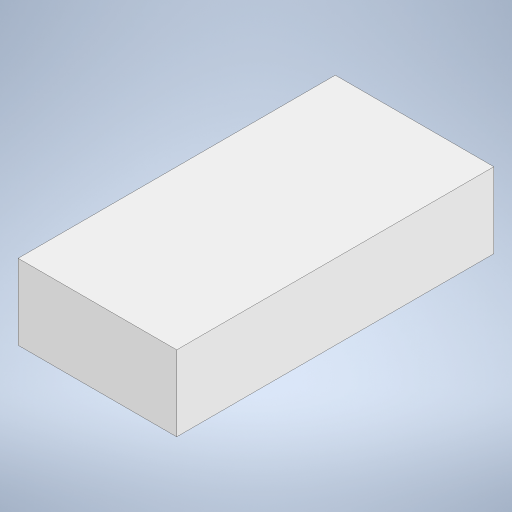
# Autodesk Inventor part: Bathtub
Saved by Autodesk Inventor 2024 (Build 280153000, 153)
## iProperties
Created: 2023-05-14
Part Number: Bathtub
Material: Generic
Document SubType Name: Modeling
Designer: Tom
Density: 1 g/cm^3
Appearance: White
Author: Tom
Autodesk Inventor part; units mm, degrees
ref_plane "YZ Plane" through (0, 0, 0) normal (1, 0, 0) x (0, 1, 0)
ref_plane "XZ Plane" through (0, 0, 0) normal (0, 1, 0) x (-1, 0, 0)
ref_plane "XY Plane" through (0, 0, 0) normal (0, 0, 1) x (1, 0, 0)
sketch "Sketch1" plane through (0, 0, 0) normal (1, 0, 0) x (0, 1, 0)
  line L0 (0, 0) -> (361.95, 0)
  line L1 (361.95, 0) -> (361.95, -1524)
  line L2 (361.95, -1524) -> (0, -1524)
  line L3 (0, -1524) -> (0, 0)
  dimension "d0" = 1524
  dimension "d2" = 361.95
  constraints: 8 end point, 2 parallel, 1 horizontal, 1 perpendicular
  measures "d0" distance of L2.end L0.start
  measures "d2" distance of L1.end L2.end
extrude "Extrusion1" add sketch "Sketch1" along normal blind 762
body "Solid1"
